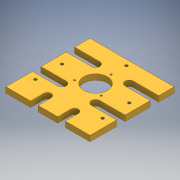
# Autodesk Inventor part: rectangularObjectiveHolder
Saved by Autodesk Inventor 2016 (Build 200138000, 138)
## iProperties
Created: 2016-03-08
Part Number: rectangularObjectiveHolder
Material: Generic
Document SubType Name: Modeling
Designer: sims01
Density: 1 g/cm^3
Appearance: Default
Author: sims01
Autodesk Inventor part; units mm, degrees
ref_plane "YZ Plane" through (0, 0, 0) normal (1, 0, 0) x (0, 1, 0)
ref_plane "XZ Plane" through (0, 0, 0) normal (0, 1, 0) x (-1, 0, 0)
ref_plane "XY Plane" through (0, 0, 0) normal (0, 0, 1) x (1, 0, 0)
sketch "Sketch1" plane through (0, 0, 0) normal (0, 0, 1) x (1, 0, 0)
  line L0 (-75, 42.5) -> (75, 42.5)
  line L1 (75, 42.5) -> (75, -107.5)
  line L2 (75, -107.5) -> (-75, -107.5)
  line L3 (-75, -107.5) -> (-75, 42.5)
  point P0 (0, 0)
  dimension "d0" = 150
  dimension "d1" = 75
  dimension "d2" = 150
  dimension "d85" = 42.5
  constraints: 8 end point, 2 parallel, 1 horizontal, 1 perpendicular
  measures "d0" distance of L0.start L0.end
  measures "d1" distance from line of point (0, 0) L1
  measures "d2" distance of L0.end L1.end
  measures "d85" distance from line of L0 point (0, 0)
extrude "baseExtrusion" add sketch "Sketch1" along normal blind 10
sketch "Sketch3" plane through (0, 0, 10) normal (0, 0, 1) x (1, 0, 0)
  circle A0 centre (0, -22.5) radius 21.25
  line L0 (-75, -107.5) -> (75, -107.5) projected
  line L1 (-75, 42.5) -> (-75, -107.5) projected
  line L2 (75, 42.5) -> (-75, 42.5) projected
  dimension "d16" = 42.5
  dimension "d68" = 75
  dimension "d84" = 65
  constraints: 1 centre point
  measures "d16" diameter of A0
  measures "d68" distance from line of A0.centre L1
  measures "d84" distance from line of A0.centre L2
extrude "objectiveExtrusion" cut sketch "Sketch3" against normal through all
sketch "Sketch5" plane through (0, 0, 10) normal (0, 0, 1) x (1, 0, 0)
  line L0 (30, 15) -> (75, 15)
  line L1 (75, 15) -> (75, 0)
  line L2 (75, 0) -> (30, 0)
  line L3 (22.5, 7.5) -> (22.5, 7.5)
  line L4 (75, -107.5) -> (75, 42.5) projected
  arc A0 (30, 15) -> (22.5, 7.5) centre (30, 7.5) ccw
  arc A1 (22.5, 7.5) -> (30, 0) centre (30, 7.5) ccw
  circle A2 centre (0, -22.5) radius 21.25 projected
  point P0 (0, 0)
  point P1 (22.5, 15)
  dimension "d34" = 15
  dimension "d35" = 7.5
  dimension "d54" = 30
  dimension "d67" = 30
  constraints: 8 end point, 4 point on circle, 4 tangent, 2 centre point, 2 parallel, 2 point on line, 1 collinear, 1 concentric, 1 horizontal, 1 perpendicular
  measures "d34" distance of L0.end L1.end
  measures "d35" radius of A0
  measures "d54" horizontal distance of A2.centre A0.centre
  measures "d67" horizontal distance of A0.centre A2.centre
extrude "cageRodBase1" cut sketch "Sketch5" against normal through all contours L0 L1 L2 A1 A0
mirror "cageRodBase2" about plane through (0, 0, 0) normal (1, 0, 0) of "cageRodBase1"
pattern_linear "cageRodBase34" count 2 spacing 60 along (0, -1, 0) of "cageRodBase1", "cageRodBase2"
sketch "Sketch8" plane through (0, 0, 0) normal (0, 0, -1) x (-1, 0, 0)
  line L0 (75, 0) -> (75, -45) projected
  line L1 (75, 15) -> (75, 42.5) projected
  circle A0 centre (0, -22.5) radius 21.25 projected
  point P0 (0, 0)
  point P1 (0, 5)
  point P2 (-23.8157, -36.25)
  point P3 (23.8157, -36.25)
  dimension "d71" = 75
  dimension "d72" = 27.5
  dimension "d75" = 360
  constraints: 4 other
  measures "d71" distance from line of L1 point (0, 5)
  measures "d72" distance of point (0, 5) A0.centre
hole "objectiveHolderMountingHoles" at (-23.8157, -36.25, 0) at (23.8157, -36.25, 0) at (0, 5, 0) direction (0, 0, 1) diameter 3.242 end through all thread size "M4x0.7" class "6H" standard "ISO Metric profile"
sketch "Sketch9" plane through (0, 0, 0) normal (0, 0, -1) x (-1, 0, 0)
  line L0 (75, -60) -> (30, -60) projected
  line L1 (30, -45) -> (75, -45) projected
  arc A0 (30, -45) -> (30, -60) centre (30, -52.5) ccw projected
  point P0 (0, 0)
  point P1 (60, -70)
  point P2 (-60, -70)
  point P3 (60, -22.5)
  point P4 (-60, -22.5)
  point P5 (0, 32.5)
  dimension "d87" = 120
  dimension "d88" = 60
  dimension "d97" = 30
  dimension "d98" = 55
  dimension "d99" = 47.5
  constraints: 3 vertical alignment, 2 horizontal alignment
  measures "d87" distance of point (-60, -70) point (60, -70)
  measures "d88" horizontal distance of point (0, 0) point (-60, -70)
  measures "d97" horizontal distance of point (60, -22.5) A0.centre
  measures "d98" vertical distance of point (0, 32.5) point (60, -22.5)
  measures "d99" distance of point (60, -22.5) point (60, -70)
hole "m6MountingHoles" at (-60, -70, 0) at (60, -70, 0) at (-60, -22.5, 0) at (60, -22.5, 0) at (0, 32.5, 0) direction (0, 0, 1) diameter 4.917 end through all counterbore diameter 10 counterbore depth 2 thread size "M6x1" class "6H" standard "ISO Metric profile"
sketch "Sketch11" plane through (0, 0, 0) normal (0, 0, -1) x (-1, 0, 0)
  line L0 (31, -107.5) -> (17.5, -107.5)
  line L1 (17.5, -107.5) -> (17.5, -84.25)
  line L2 (24.25, -77.5) -> (24.25, -77.5)
  line L3 (31, -84.25) -> (31, -107.5)
  line L4 (-75, -107.5) -> (75, -107.5) projected
  arc A0 (31, -84.25) -> (24.25, -77.5) centre (24.25, -84.25) ccw
  arc A1 (24.25, -77.5) -> (17.5, -84.25) centre (24.25, -84.25) ccw
  point P0 (0, 0)
  point P1 (17.5, -77.5)
  dimension "d110" = 13.5
  dimension "d111" = 30
  dimension "d112" = 6.75
  dimension "d113" = 6.75
  dimension "d114" = 24.25
  constraints: 8 end point, 4 point on circle, 4 tangent, 2 centre point, 2 parallel, 2 point on line, 1 collinear, 1 horizontal, 1 perpendicular
  measures "d110" distance between parallel lines of L1 L3
  measures "d111" distance of L0.end point (17.5, -77.5)
  measures "d112" radius of A0
  measures "d113" radius of A1
  measures "d114" horizontal distance of point (0, 0) A0.centre
extrude "filterWheelPost1" cut sketch "Sketch11" against normal through all
mirror "filterWheelPost2" about plane through (0, 0, 0) normal (1, 0, 0) of "filterWheelPost1"
equation "\"d1\" = 0.5 * d0"
equation "\"d68\" = 0.5 * d0"
equation "\"d71\" = d68"
equation "\"d88\" = 0.5 * d87"
body "Solid1"
